GridUp-Kutu (Autodesk Fusion 360 design; units mm, degrees)
part number: 2026-09-14-07-36-03-763
Autodesk Fusion 360 part; units mm, degrees
sketch "Çizim53" plane through (0, 0, 0) normal (0, 0, 1) x (1, 0, 0)
  line L0 (0, 0) -> (120, 0)
  line L1 (120, 0) -> (120, 80)
  line L2 (120, 80) -> (0, 80)
  line L3 (0, 80) -> (0, 0)
extrude "Ekstrüzyon53" add sketch "Çizim53" along normal blind 46 makes body 1
fillet "Kavis7" radius 4 4 edges at (0, 80, 23) (120, 80, 23) (120, 0, 23) (0, 0, 23) on bodies 1
shell "Kabuk4" thickness 2 removed faces 1 at (78.6667, 26.6667, 46) on bodies 1
sketch "Çizim54" plane through (0, 0, 0) normal (0, 0, 1) x (1, 0, 0)
  circle A0 centre (5, 5) radius 3.5
  circle A1 centre (115, 5) radius 3.5
  circle A2 centre (5, 75) radius 3.5
  circle A3 centre (115, 75) radius 3.5
extrude "Ekstrüzyon54" add sketch "Çizim54" along normal blind 46 bodies 1
sketch "Çizim55" plane through (0, 0, 0) normal (0, 0, 1) x (1, 0, 0)
  circle A0 centre (12, 12) radius 3
  circle A1 centre (108, 12) radius 3
  circle A2 centre (12, 68) radius 3
  circle A3 centre (108, 68) radius 3
extrude "Ekstrüzyon55" add sketch "Çizim55" along normal blind 39.4 bodies 1
ref_plane "WorkPlane15" through (0, 0, 39.4) normal (0, 0, 1) x (1, 0, 0)
sketch "Çizim56" plane through (0, 0, 39.4) normal (0, 0, 1) x (1, 0, 0)
  circle A0 centre (12, 12) radius 1.25
  circle A1 centre (108, 12) radius 1.25
  circle A2 centre (12, 68) radius 1.25
  circle A3 centre (108, 68) radius 1.25
extrude "Ekstrüzyon56" cut sketch "Çizim56" against normal blind 8 bodies 1
ref_plane "WorkPlane16" through (0, 0, 46) normal (0, 0, 1) x (1, 0, 0)
sketch "Çizim57" plane through (0, 0, 46) normal (0, 0, 1) x (1, 0, 0)
  line L0 (0, 0) -> (120, 0)
  line L1 (120, 0) -> (120, 80)
  line L2 (120, 80) -> (0, 80)
  line L3 (0, 80) -> (0, 0)
extrude "Ekstrüzyon57" add sketch "Çizim57" along normal blind 4 separate body makes body 2
fillet "Kavis8" radius 4 4 edges at (0, 80, 48) (120, 80, 48) (120, 0, 48) (0, 0, 48) on bodies 2
ref_plane "WorkPlane17" through (0, 0, 50) normal (0, 0, 1) x (1, 0, 0)
sketch "Çizim58" plane through (0, 0, 50) normal (0, 0, 1) x (1, 0, 0)
  circle A0 centre (60, 42.5) radius 11.5
extrude "Ekstrüzyon58" add sketch "Çizim58" along normal blind 2 bodies 2
sketch "Çizim59" plane through (0, 0, 50) normal (0, 0, 1) x (1, 0, 0)
  circle A0 centre (60, 42.5) radius 7.5
extrude "Ekstrüzyon59" cut sketch "Çizim59" along normal mid plane 16 bodies 2
chamfer "Pah4" distance 3 angle 45 1 edges at (53.0075, 45.2121, 52) on bodies 2
sketch "Çizim60" plane through (0, 0, 50) normal (0, 0, 1) x (1, 0, 0)
  circle A0 centre (12, 36) radius 4.5
extrude "Ekstrüzyon60" add sketch "Çizim60" along normal blind 1.5 bodies 2
sketch "Çizim61" plane through (0, 0, 50) normal (0, 0, 1) x (1, 0, 0)
  circle A0 centre (12, 36) radius 3.25
extrude "Ekstrüzyon61" cut sketch "Çizim61" along normal mid plane 16 bodies 2
sketch "Çizim62" plane through (0, 0, 50) normal (0, 0, 1) x (1, 0, 0)
  circle A0 centre (30, 70) radius 1.6
extrude "Ekstrüzyon62" cut sketch "Çizim62" along normal mid plane 16 bodies 2
sketch "Çizim63" plane through (0, 0, 50) normal (0, 0, 1) x (1, 0, 0)
  circle A0 centre (5, 5) radius 1.6
  circle A1 centre (115, 5) radius 1.6
  circle A2 centre (5, 75) radius 1.6
  circle A3 centre (115, 75) radius 1.6
extrude "Ekstrüzyon63" cut sketch "Çizim63" along normal mid plane 16 bodies 2
sketch "Çizim64" plane through (0, 0, 50) normal (0, 0, 1) x (1, 0, 0)
  circle A0 centre (5, 5) radius 1.25
  circle A1 centre (115, 5) radius 1.25
  circle A2 centre (5, 75) radius 1.25
  circle A3 centre (115, 75) radius 1.25
extrude "Ekstrüzyon64" cut sketch "Çizim64" against normal blind 16 bodies 1
ref_plane "WorkPlane18" through (0, 0, 47.5) normal (0, 0, 1) x (1, 0, 0)
sketch "Çizim65" plane through (0, 0, 47.5) normal (0, 0, 1) x (1, 0, 0)
  circle A0 centre (60, 42.5) radius 7.5
extrude "Ekstrüzyon65" add sketch "Çizim65" along normal mid plane 1 separate body makes body 3
sketch "Çizim66" plane through (0, 0, 0) normal (0, 1, 0) x (1, 0, 0)
  circle A0 centre (17.5, -23) radius 6.25
  circle A1 centre (40, -23) radius 3.2
  circle A2 centre (65, -23) radius 6.25
  circle A3 centre (102.5, -23) radius 6.25
extrude "Ekstrüzyon66" cut sketch "Çizim66" along normal mid plane 6 bodies 1
sketch "Çizim67" plane through (0, 0, 0) normal (0, 0, 1) x (1, 0, 0)
  line L0 (12.75, 42.5) -> (22.25, 42.5)
  arc A0 (22.25, 42.5) -> (22.25, 48) centre (22.25, 45.25) ccw
  line L1 (22.25, 48) -> (12.75, 48)
  arc A1 (12.75, 48) -> (12.75, 42.5) centre (12.75, 45.25) ccw
  line L2 (97.75, 42.5) -> (107.25, 42.5)
  arc A2 (107.25, 42.5) -> (107.25, 48) centre (107.25, 45.25) ccw
  line L3 (107.25, 48) -> (97.75, 48)
  arc A3 (97.75, 48) -> (97.75, 42.5) centre (97.75, 45.25) ccw
extrude "Ekstrüzyon67" cut sketch "Çizim67" along normal mid plane 6 bodies 1
sketch "Çizim68" plane through (0, 0, 0) normal (0, 0, 1) x (1, 0, 0)
  circle A0 centre (7.5, 7.5) radius 3.5
  circle A1 centre (112.5, 7.5) radius 3.5
  circle A2 centre (7.5, 72.5) radius 3.5
  circle A3 centre (112.5, 72.5) radius 3.5
extrude "Ekstrüzyon68" cut sketch "Çizim68" along normal mid plane 2 bodies 1
sketch "Çizim69" plane through (0, 0, 0) normal (0, 0, 1) x (1, 0, 0)
  line L0 (42.5, 20) -> (77.5, 20)
  line L1 (77.5, 20) -> (77.5, 62)
  line L2 (77.5, 62) -> (42.5, 62)
  line L3 (42.5, 62) -> (42.5, 20)
extrude "Ekstrüzyon69" add sketch "Çizim69" against normal blind 5 separate body makes body 4
ref_plane "WorkPlane19" through (0, 0, -5) normal (0, 0, 1) x (1, 0, 0)
sketch "Çizim70" plane through (0, 0, -5) normal (0, 0, 1) x (1, 0, 0)
  line L0 (42.5, 23.25) -> (77.5, 23.25)
  line L1 (77.5, 23.25) -> (77.5, 58.75)
  line L2 (77.5, 58.75) -> (42.5, 58.75)
  line L3 (42.5, 58.75) -> (42.5, 23.25)
extrude "Ekstrüzyon70" cut sketch "Çizim70" along normal mid plane 6 bodies 4
equation "d162 = -( 8 mm )"
equation "d185 = -( 16 mm )"
equation "d197 = -( 5 mm )"
named bodies: "Gövde", "Kapak", "IR pencere", "DIN klips"
